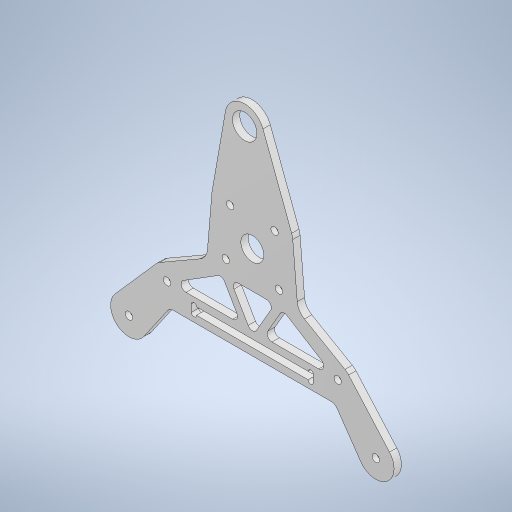
# Autodesk Inventor part: 中間ユニット内
Saved by Autodesk Inventor 2023 (Build 270158000, 158)
## iProperties
Created: 2022-03-07
Part Number: 中間ユニット内
Material: Aluminum 2014-T6
Document SubType Name: Modeling
Designer: acps
Density: 2.78927 g/cm^3
Appearance: Satin
Author: acps
Autodesk Inventor part; units mm, degrees
ref_plane "YZ Plane" through (0, 0, 0) normal (1, 0, 0) x (0, 1, 0)
ref_plane "XZ Plane" through (0, 0, 0) normal (0, 1, 0) x (-1, 0, 0)
ref_plane "XY Plane" through (0, 0, 0) normal (0, 0, 1) x (1, 0, 0)
sketch "Sketch2" plane through (0, 0, 0) normal (0, 0, 1) x (1, 0, 0)
  line L0 (0, 0) -> (0, 5.2095) construction
  circle A0 centre (0, 29.1078) radius 6.7008 construction
  arc A1 (-5.7731, 13.9993) -> (-7.5051, 10.9993) centre (-5.7731, 11.9993) ccw
  line L1 (-5.7731, 13.9993) -> (5.7731, 13.9993)
  arc A2 (7.5051, 10.9993) -> (5.7731, 13.9993) centre (5.7731, 11.9993) ccw
  line L2 (-7.5051, 10.9993) -> (-1.7321, 1)
  line L3 (7.5051, 10.9993) -> (1.7321, 1)
  arc A3 (-1.7321, 1) -> (1.7321, 1) centre (0, 2) ccw
  line L4 (-25, -4.5) -> (25, -4.5) construction
  line L5 (-23.95, -3) -> (-23.95, -6) construction
  line L6 (-25, -3) -> (-25, -6)
  line L7 (-22.9, -6) -> (-22.9, -3) construction
  arc A4 (-22.9, -3) -> (-25, -3) centre (-23.95, -3) ccw
  arc A5 (-25, -6) -> (-22.9, -6) centre (-23.95, -6) ccw
  arc A6 (25, -3) -> (22.9, -3) centre (23.95, -3) ccw
  line L8 (25, -3) -> (25, -6)
  arc A7 (22.9, -6) -> (25, -6) centre (23.95, -6) ccw
  line L9 (14.204, 12.4682) -> (28.2856, 3.6976)
  arc A8 (27.2282, 0) -> (28.2856, 3.6976) centre (27.2282, 2) ccw
  line L10 (27.2282, 0) -> (8.0829, 0)
  line L11 (-25, -3) -> (-23.95, -3) construction
  line L12 (-22.9, -3) -> (22.9, -3)
  line L13 (-25, -6) -> (-23.95, -6) construction
  line L14 (-22.9, -6) -> (22.9, -6)
  line L15 (-26.5636, -1.95) -> (-22.5758, -1.95) construction
  circle A9 centre (9.1116, 40) radius 4.5 construction
  circle A10 centre (9.1116, 40) radius 1.5
  circle A11 centre (10.8954, 20) radius 4.5 construction
  circle A12 centre (10.8954, 20) radius 1.5
  circle A13 centre (50.6355, -20) radius 4.5 construction
  circle A14 centre (50.6355, -20) radius 1.5
  line L16 (32.3294, -9) -> (0, -9)
  circle A15 centre (-9.1116, 40) radius 4.5 construction
  circle A16 centre (-9.1116, 40) radius 1.5
  circle A17 centre (-10.8954, 20) radius 4.5 construction
  circle A18 centre (-10.8954, 20) radius 1.5
  line L17 (-14.204, 12.4682) -> (-28.2856, 3.6976)
  line L18 (-27.2282, 0) -> (-8.0829, 0)
  arc A19 (-28.2856, 3.6976) -> (-27.2282, 0) centre (-27.2282, 2) ccw
  line L19 (-32.3294, -9) -> (0, -9)
  arc A20 (14.204, 12.4682) -> (11.4146, 11.7706) centre (13.1466, 10.7706) ccw
  line L20 (11.4146, 11.7706) -> (6.3509, 3)
  arc A21 (6.3509, 3) -> (8.0829, 0) centre (8.0829, 2) ccw
  arc A22 (-11.4146, 11.7706) -> (-14.204, 12.4682) centre (-13.1466, 10.7706) ccw
  line L21 (-11.4146, 11.7706) -> (-6.3509, 3)
  arc A23 (-8.0829, 0) -> (-6.3509, 3) centre (-8.0829, 2) ccw
  circle A24 centre (10.8954, 20) radius 7.5
  circle A25 centre (9.1116, 40) radius 7.5
  line L22 (16.5836, 40.6477) -> (18.4178, 19.4897)
  arc A26 (18.4178, 19.4897) -> (21.3954, 14.8117) centre (24.3954, 20.0079) ccw
  line L23 (21.3954, 14.8117) -> (38.0125, 5.2178)
  circle A27 centre (50.6355, -20) radius 7.5
  line L24 (9.1116, 47.5) -> (0, 47.5)
  line L25 (-9.1116, 47.5) -> (0, 47.5)
  circle A28 centre (-9.1116, 40) radius 7.5
  line L26 (-16.5836, 40.6477) -> (-18.4178, 19.4897)
  circle A29 centre (-10.8954, 20) radius 7.5
  circle A30 centre (-50.6355, -20) radius 7.5
  line L27 (-32.3294, -9) -> (0, -9)
  circle A31 centre (-50.6355, -20) radius 4.5 construction
  circle A32 centre (-50.6355, -20) radius 1.5
  arc A33 (-21.3954, 14.8117) -> (-18.4178, 19.4897) centre (-24.3954, 20.0079) ccw
  circle A34 centre (35, 0) radius 1.5
  circle A35 centre (35, 0) radius 3.025
  circle A36 centre (35, 0) radius 6.025
  line L28 (-21.3954, 14.8117) -> (-38.0125, 5.2178)
  circle A37 centre (-35, 0) radius 6.025
  circle A38 centre (-35, 0) radius 3.025
  circle A39 centre (-35, 0) radius 1.5
  circle A40 centre (9.1116, 40) radius 3.025
  circle A41 centre (10.8954, 20) radius 3.025
  circle A42 centre (50.6355, -20) radius 3.025
  circle A43 centre (-9.1116, 40) radius 3.025
  circle A44 centre (-10.8954, 20) radius 3.025
  circle A45 centre (-50.6355, -20) radius 3.025
  line L29 (56.2658, -15.0452) -> (39.523, 3.9803)
  line L30 (-56.2658, -15.0452) -> (-39.523, 3.9803)
  line L31 (-20.812, -60) -> (26.178, -60)
  circle A46 centre (-3.14, 71) radius 5.025
  circle A47 centre (-3.14, 71) radius 8.025
  line L32 (-11.0443, 72.3867) -> (-16.4988, 41.296)
  line L33 (4.3688, 73.8317) -> (16.1292, 42.6464)
  arc A48 (34.7962, -10.2927) -> (32.3294, -9) centre (32.3294, -12) ccw
  line L34 (34.7962, -10.2927) -> (44.4684, -24.2681)
  line L35 (-34.7962, -10.2927) -> (-44.4684, -24.2681)
  arc A49 (-32.3294, -9) -> (-34.7962, -10.2927) centre (-32.3294, -12) ccw
  circle A50 centre (0, 29.1078) radius 4.7008
  point P0 (-23.95, -4.5)
  point P1 (0, 0)
  point P2 (-39.523, 3.9803)
  dimension "d328" = 2
  dimension "d329" = 2
  dimension "d330" = 30
  dimension "d331" = 2
  dimension "d332" = 50
  dimension "d333" = 3
  dimension "d334" = 2.1
  dimension "d335" = 25
  dimension "d336" = 2
  dimension "d337" = 60
  dimension "d338" = 3
  dimension "d339" = 2
  dimension "d340" = 2
  dimension "d341" = 3
  dimension "d342" = 3
  dimension "d343" = 3
  dimension "d344" = 6
  dimension "d345" = 3
  dimension "d346" = 3
  dimension "d347" = 6.05
  dimension "d348" = 3
  dimension "d349" = 30
  dimension "d350" = 6.05
  dimension "d351" = 6.05
  dimension "d352" = 6.05
  dimension "d353" = 60
  dimension "d354" = 10.05
  dimension "d355" = 71
  dimension "d356" = 3.14
  dimension "d357" = 3
  dimension "d358" = 4.5
  dimension "d359" = 3
  dimension "d360" = 2
  constraints: 74 end point, 51 centre point, 48 point on circle, 41 symmetric about line, 38 tangent, 7 coincident, 7 horizontal, 6 parallel, 3 midpoint, 2 point on line, 2 vertical, 1 horizontal alignment, 1 vertical alignment, 34 other
  measures "d328" radius of A2
  measures "d329" radius of A3
  measures "d330" angle of L0 L2
  measures "d331" radius of A1
  measures "d332" distance of L4.start L4.end
  measures "d333" distance of L5.start L5.end
  measures "d334" diameter of A5
  measures "d335" horizontal distance of point (-25, -4.5) L0.start
  measures "d336" radius of A8
  measures "d337" angle of L2 L3
  measures "d338" distance between parallel lines of L16 L14
  measures "d339" radius of A20
  measures "d340" radius of A21
  measures "d341" distance between parallel lines of L3 L20
  measures "d342" radial gap between concentric circles of A11 A24
  measures "d343" radial gap between concentric circles of A9 A25
  measures "d344" radius of A26
  measures "d345" radial gap between concentric circles of A13 A27
  measures "d346" diameter of A34
  measures "d347" diameter of A35
  measures "d348" radial gap between concentric circles of A35 A36
  measures "d349" angle of L10 L23
  measures "d350" diameter of A40
  measures "d351" diameter of A41
  measures "d352" diameter of A42
  measures "d353" distance from line of point (0, 0) L31
  measures "d354" diameter of A46
  measures "d355" vertical distance of L0.start A46.centre
  measures "d356" horizontal distance of L0.start A46.centre
  measures "d357" radial gap between concentric circles of A46 A47
  measures "d358" distance from line of L4 L0.start
  measures "d359" radius of A48
  measures "d360" radial gap between concentric circles of A50 A0
extrude "Extrusion7" add sketch "Sketch2" against normal blind 3 contours A1 A29 L26 A28 L25 L24 A25 L22 A24 A2 L1 | A1 L2 A3 L3 A2 A24 A20 L20 A21 L10 A8 A36 L29 A27 L34 A48 L16 L19 A49 L35 A30 L30 A37 A19 L18 A23 L21 A22 A29 | A29 L26 | A22 L17 A19 A37 L28 A33 L26 A29 | A24 L22 | A24 L22 A26 L23 A36 A8 L9 A20 | A28 | A25 | A37 | L32 A47 L33 A25 L24 L25 A28 | A47 | A36 | A30 | A27 picked at (-4.991, 20.8477) picked at (7.0332, 24.545)
extrude "Extrusion8" add sketch "Sketch2" against normal blind 2 contours A35 | A38 | A40 | A41 | A42 | A43 | A44 | A45
body "Solid4"
